Autodesk Fusion 360 part; units mm, degrees
(part 5 of 5)
sketch "Sketch25" plane through (0.7254, 0, 5.7707) normal (0.12473, 0, 0.992191) x (0, 1, 0)
  line L0 (293.4635, 73.8171) -> (293.4635, 58.6434)
  arc A0 (292.1232, 54.8991) -> (293.4635, 58.6434) centre (287.5635, 58.6434) ccw
  line L1 (292.1232, 54.8991) -> (275.8299, 35.0581)
  arc A1 (273.8014, 33.6658) -> (275.8299, 35.0581) centre (272.4102, 37.8664) ccw
  line L2 (273.8014, 33.6658) -> (261.9665, 29.7462)
  arc A2 (258.1218, 32.1079) -> (261.9665, 29.7462) centre (261.039, 32.5466) ccw
  line L3 (258.1218, 32.1079) -> (254.2531, 57.8338)
  arc A3 (256.0736, 63.8745) -> (254.2531, 57.8338) centre (261.5461, 58.9306) ccw
  line L4 (256.0736, 63.8745) -> (269.2803, 78.4929)
  arc A4 (277.0376, 80.9788) -> (269.2803, 78.4929) centre (275.3, 73.0546) ccw
  line L5 (277.0376, 80.9788) -> (289.9863, 78.1394)
  arc A5 (293.4635, 73.8171) -> (289.9863, 78.1394) centre (289.0385, 73.8171) ccw
  line L6 (230.7717, 93.4693) -> (226.5548, 85.749)
  arc A6 (222.0059, 84.0707) -> (226.5548, 85.749) centre (223.3186, 87.5166) ccw
  line L7 (222.0059, 84.0707) -> (215.7224, 86.4644)
  arc A7 (214.1574, 90.5861) -> (215.7224, 86.4644) centre (216.7726, 89.2211) ccw
  line L8 (214.1574, 90.5861) -> (217.2044, 96.4242)
  arc A8 (220.6389, 100.0016) -> (217.2044, 96.4242) centre (225.0501, 92.3293) ccw
  line L9 (220.6389, 100.0016) -> (226.4521, 103.3439)
  arc A9 (230.7073, 101.7599) -> (226.4521, 103.3439) centre (227.9225, 100.7865) ccw
  line L10 (230.7073, 101.7599) -> (231.3102, 100.0349)
  arc A10 (230.7717, 93.4693) -> (231.3102, 100.0349) centre (223.6521, 97.3581) ccw
  arc A11 (211.2158, 50.6501) -> (212.3403, 56.2234) centre (209.4758, 53.9013) ccw
  line L11 (211.2158, 50.6501) -> (201.0039, 45.1846)
  arc A12 (196.7325, 47.1438) -> (201.0039, 45.1846) centre (199.6118, 47.7855) ccw
  line L12 (196.7325, 47.1438) -> (190.7528, 73.975)
  arc A13 (195.9237, 76.4744) -> (190.7528, 73.975) centre (193.6321, 74.6167) ccw
  line L13 (195.9237, 76.4744) -> (212.3403, 56.2234)
  arc A14 (133.0891, 19.5942) -> (135.5665, 15.0427) centre (135.5665, 17.9927) ccw
  line L14 (133.0891, 19.5942) -> (153.5813, 51.294)
  arc A15 (157.3818, 52.3291) -> (153.5813, 51.294) centre (156.0587, 49.6924) ccw
  line L15 (157.3818, 52.3291) -> (171.2495, 45.3704)
  arc A16 (175.2679, 40.8003) -> (171.2495, 45.3704) centre (167.6111, 38.1196) ccw
  line L16 (175.2679, 40.8003) -> (182.9119, 18.9675)
  arc A17 (180.1276, 15.0427) -> (182.9119, 18.9675) centre (180.1276, 17.9927) ccw
  line L17 (180.1276, 15.0427) -> (135.5665, 15.0427)
  line L18 (123.35, 103.697) -> (120.1949, 82.505)
  arc A18 (115.2719, 78.7654) -> (120.1949, 82.505) centre (115.8182, 83.1566) ccw
  line L19 (115.2719, 78.7654) -> (87.1104, 82.2687)
  arc A19 (83.9707, 86.7489) -> (87.1104, 82.2687) centre (87.5657, 85.928) ccw
  line L20 (83.9707, 86.7489) -> (88.0477, 104.6024)
  arc A20 (92.2179, 107.9276) -> (88.0477, 104.6024) centre (92.2179, 103.6501) ccw
  line L21 (92.2179, 107.9276) -> (119.7027, 107.9276)
  arc A21 (123.35, 103.697) -> (119.7027, 107.9276) centre (119.7027, 104.2401) ccw
  line L22 (85.4902, 103.2388) -> (81.1941, 84.4262)
  arc A22 (79.0443, 81.4437) -> (81.1941, 84.4262) centre (76.5925, 85.477) ccw
  line L23 (79.0443, 81.4437) -> (65.0016, 72.9802)
  arc A23 (62.0516, 72.6514) -> (65.0016, 72.9802) centre (63.1527, 76.1707) ccw
  line L24 (62.0516, 72.6514) -> (12.6248, 88.1163)
  arc A24 (10.1419, 91.4948) -> (12.6248, 88.1163) centre (13.6819, 91.4948) ccw
  line L25 (10.1419, 91.4948) -> (10.1419, 100.0343)
  arc A25 (13.5344, 103.4268) -> (10.1419, 100.0343) centre (13.5344, 100.0343) ccw
  line L26 (13.5344, 103.4268) -> (37.6527, 103.4268)
  line L27 (37.6527, 103.4268) -> (42.657, 107.9276)
  line L28 (42.657, 107.9276) -> (81.7514, 107.9276)
  arc A26 (85.4902, 103.2388) -> (81.7514, 107.9276) centre (81.7514, 104.0926) ccw
  arc A27 (103.6411, 44.2546) -> (107.543, 46.9984) centre (104.5933, 47.0467) ccw
  line L29 (103.6411, 44.2546) -> (75.7593, 53.7636)
  arc A28 (71.4916, 57.5515) -> (75.7593, 53.7636) centre (78.1398, 60.7438) ccw
  line L30 (71.4916, 57.5515) -> (66.9703, 66.9675)
  arc A29 (68.665, 72.6667) -> (66.9703, 66.9675) centre (70.9592, 68.8829) ccw
  line L31 (68.665, 72.6667) -> (79.3035, 79.1172)
  arc A30 (85.3097, 80.4194) -> (79.3035, 79.1172) centre (84.1979, 71.0451) ccw
  line L32 (85.3097, 80.4194) -> (105.004, 78.0835)
  arc A31 (107.9965, 74.659) -> (105.004, 78.0835) centre (104.6045, 74.7146) ccw
  line L33 (107.9965, 74.659) -> (107.543, 46.9984)
  line L34 (77.6309, 51.2153) -> (106.5409, 41.2402)
  arc A32 (108.7653, 39.733) -> (106.5409, 41.2402) centre (104.857, 36.36) ccw
  line L35 (108.7653, 39.733) -> (125.8648, 19.9201)
  arc A33 (123.6315, 15.0427) -> (125.8648, 19.9201) centre (123.6315, 17.9927) ccw
  line L36 (123.6315, 15.0427) -> (71.6211, 15.0427)
  arc A34 (67.2556, 20.1909) -> (71.6211, 15.0427) centre (71.6211, 19.4677) ccw
  line L37 (67.2556, 20.1909) -> (71.8221, 47.7555)
  arc A35 (77.6309, 51.2153) -> (71.8221, 47.7555) centre (76.1876, 47.0323) ccw
  arc A36 (213.8317, 57.7017) -> (217.428, 56.9204) centre (216.1194, 59.5643) ccw
  line L38 (213.8317, 57.7017) -> (196.1913, 79.369)
  arc A37 (198.0965, 84.1566) -> (196.1913, 79.369) centre (198.479, 81.2315) ccw
  line L39 (198.0965, 84.1566) -> (208.6237, 85.5329)
  arc A38 (213.4569, 85.0107) -> (208.6237, 85.5329) centre (209.9622, 75.2951) ccw
  line L40 (213.4569, 85.0107) -> (222.0557, 81.9177)
  arc A39 (226.309, 78.3859) -> (222.0557, 81.9177) centre (219.3099, 74.284) ccw
  line L41 (226.309, 78.3859) -> (232.4628, 67.8857)
  arc A40 (231.2263, 63.7503) -> (232.4628, 67.8857) centre (229.9177, 66.3941) ccw
  line L42 (231.2263, 63.7503) -> (217.428, 56.9204)
  line L43 (249.3606, 15.0427) -> (236.4115, 15.0427)
  arc A41 (232.5299, 17.3431) -> (236.4115, 15.0427) centre (236.4115, 19.4677) ccw
  line L44 (232.5299, 17.3431) -> (215.1327, 49.1283)
  arc A42 (216.7158, 54.1958) -> (215.1327, 49.1283) centre (218.3674, 50.8988) ccw
  line L45 (216.7158, 54.1958) -> (232.339, 62.0219)
  arc A43 (239.2829, 63.0131) -> (232.339, 62.0219) centre (237.2937, 52.1309) ccw
  line L46 (239.2829, 63.0131) -> (248.8594, 61.2625)
  arc A44 (252.4432, 57.5422) -> (248.8594, 61.2625) centre (248.0637, 56.9097) ccw
  line L47 (252.4432, 57.5422) -> (256.3019, 30.8271)
  arc A45 (255.7697, 24.7696) -> (256.3019, 30.8271) centre (243.1633, 28.9294) ccw
  line L48 (255.7697, 24.7696) -> (253.5627, 18.0811)
  arc A46 (249.3606, 15.0427) -> (253.5627, 18.0811) centre (249.3606, 19.4677) ccw
  line L49 (293.4635, 103.5026) -> (293.4635, 84.9001)
  arc A47 (287.9958, 80.5997) -> (293.4635, 84.9001) centre (289.0385, 84.9001) ccw
  line L50 (287.9958, 80.5997) -> (274.4552, 83.8829)
  arc A48 (272.2404, 86.2656) -> (274.4552, 83.8829) centre (275.1504, 86.7498) ccw
  line L51 (272.2404, 86.2656) -> (269.4929, 102.7762)
  arc A49 (273.8579, 107.9276) -> (269.4929, 102.7762) centre (273.8579, 103.5026) ccw
  line L52 (273.8579, 107.9276) -> (289.0385, 107.9276)
  arc A50 (293.4635, 103.5026) -> (289.0385, 107.9276) centre (289.0385, 103.5026) ccw
  line L53 (290.9668, 32.2801) -> (281.6207, 33.491)
  arc A51 (280.1951, 37.0893) -> (281.6207, 33.491) centre (281.9049, 35.6851) ccw
  line L54 (280.1951, 37.0893) -> (289.5412, 48.4704)
  arc A52 (293.4635, 47.0663) -> (289.5412, 48.4704) centre (291.251, 47.0663) ccw
  arc A53 (290.9668, 32.2801) -> (293.4635, 34.4743) centre (291.251, 34.4743) ccw
  line L55 (233.851, 98.8529) -> (232.3424, 102.9719)
  arc A54 (235.8049, 107.9276) -> (232.3424, 102.9719) centre (235.8049, 104.2401) ccw
  line L56 (235.8049, 107.9276) -> (262.6115, 107.9276)
  arc A55 (266.9865, 104.166) -> (262.6115, 107.9276) centre (262.6115, 103.5026) ccw
  line L57 (266.9865, 104.166) -> (268.8676, 91.7606)
  arc A56 (264.0999, 87.6951) -> (268.8676, 91.7606) centre (265.2218, 91.2078) ccw
  line L58 (264.0999, 87.6951) -> (236.1917, 96.6084)
  arc A57 (233.851, 98.8529) -> (236.1917, 96.6084) centre (237.3135, 100.1211) ccw
  line L59 (201.7431, 17.6617) -> (199.3291, 39.0432)
  arc A58 (201.6545, 43.4497) -> (199.3291, 39.0432) centre (203.7262, 39.5396) ccw
  line L60 (201.6545, 43.4497) -> (210.1198, 47.9348)
  arc A59 (214.0829, 46.7549) -> (210.1198, 47.9348) centre (211.5009, 45.3281) ccw
  line L61 (214.0829, 46.7549) -> (229.1883, 19.4195)
  arc A60 (226.6063, 15.0427) -> (229.1883, 19.4195) centre (226.6063, 17.9927) ccw
  line L62 (226.6063, 15.0427) -> (204.6745, 15.0427)
  arc A61 (201.7431, 17.6617) -> (204.6745, 15.0427) centre (204.6745, 17.9927) ccw
  arc A62 (156.4587, 58.9806) -> (157.4975, 54.5636) centre (158.8136, 57.2038) ccw
  line L63 (156.4587, 58.9806) -> (176.5219, 85.5722)
  arc A63 (182.035, 86.864) -> (176.5219, 85.5722) centre (180.0543, 82.9071) ccw
  line L64 (182.035, 86.864) -> (183.2206, 86.2706)
  arc A64 (187.1226, 81.2581) -> (183.2206, 86.2706) centre (179.9194, 79.6756) ccw
  line L65 (187.1226, 81.2581) -> (194.4335, 47.9794)
  arc A65 (191.3482, 44.4035) -> (194.4335, 47.9794) centre (191.5522, 47.3464) ccw
  line L66 (191.3482, 44.4035) -> (178.6355, 45.2846)
  arc A66 (173.0748, 46.7985) -> (178.6355, 45.2846) centre (179.6553, 59.9993) ccw
  line L67 (173.0748, 46.7985) -> (157.4975, 54.5636)
  line L68 (121.5744, 78.7404) -> (125.6327, 105.4212)
  arc A67 (128.5492, 107.9276) -> (125.6327, 105.4212) centre (128.5492, 104.9776) ccw
  line L69 (128.5492, 107.9276) -> (172.3385, 107.9276)
  arc A68 (175.2618, 105.3735) -> (172.3385, 107.9276) centre (172.3385, 104.9776) ccw
  line L70 (175.2618, 105.3735) -> (177.1399, 91.508)
  arc A69 (176.2747, 88.2323) -> (177.1399, 91.508) centre (172.7549, 90.914) ccw
  line L71 (176.2747, 88.2323) -> (152.619, 57.1839)
  arc A70 (146.4088, 56.3524) -> (152.619, 57.1839) centre (149.0992, 59.8656) ccw
  line L72 (146.4088, 56.3524) -> (123.5394, 73.8653)
  arc A71 (121.5744, 78.7404) -> (123.5394, 73.8653) centre (126.6782, 77.9641) ccw
  line L73 (64.1302, 68.3113) -> (70.1435, 55.2951)
  arc A72 (70.492, 52.7161) -> (70.1435, 55.2951) centre (66.1265, 53.4393) ccw
  line L74 (70.492, 52.7161) -> (64.7618, 18.1275)
  arc A73 (61.1239, 15.0427) -> (64.7618, 18.1275) centre (61.1239, 18.7302) ccw
  line L75 (61.1239, 15.0427) -> (53.0443, 15.0427)
  arc A74 (50.5643, 16.3952) -> (53.0443, 15.0427) centre (53.0443, 17.9927) ccw
  line L76 (50.5643, 16.3952) -> (10.9643, 77.8757)
  arc A75 (10.1419, 80.6712) -> (10.9643, 77.8757) centre (15.3044, 80.6712) ccw
  line L77 (10.1419, 80.6712) -> (10.1419, 82.7029)
  arc A76 (13.9723, 85.5184) -> (10.1419, 82.7029) centre (13.0919, 82.7029) ccw
  line L78 (13.9723, 85.5184) -> (61.4337, 70.6789)
  arc A77 (64.1302, 68.3113) -> (61.4337, 70.6789) centre (60.1132, 66.4555) ccw
  arc A78 (10.1419, 18.7302) -> (13.8294, 15.0427) centre (13.8294, 18.7302) ccw
  line L79 (10.1419, 18.7302) -> (10.1419, 65.1989)
  arc A79 (15.5677, 66.8029) -> (10.1419, 65.1989) centre (13.0919, 65.1989) ccw
  line L80 (15.5677, 66.8029) -> (45.4146, 20.7352)
  arc A80 (42.3199, 15.0427) -> (45.4146, 20.7352) centre (42.3199, 18.7302) ccw
  line L81 (42.3199, 15.0427) -> (13.8294, 15.0427)
  arc A81 (127.0398, 21.5138) -> (131.7372, 21.8193) centre (129.273, 23.4413) ccw
  line L82 (127.0398, 21.5138) -> (111.2377, 39.8234)
  arc A82 (109.448, 44.8203) -> (111.2377, 39.8234) centre (116.8209, 44.642) ccw
  line L83 (109.448, 44.8203) -> (110.1305, 73.0437)
  arc A83 (116.5331, 76.1094) -> (110.1305, 73.0437) centre (114.1118, 72.9475) ccw
  line L84 (116.5331, 76.1094) -> (147.6751, 52.2615)
  arc A84 (148.5132, 47.3064) -> (147.6751, 52.2615) centre (145.4331, 49.3338) ccw
  line L85 (148.5132, 47.3064) -> (131.7372, 21.8193)
  arc A85 (188.1391, 86.2233) -> (194.2757, 85.4006) centre (192.6185, 96.3383) ccw
  line L86 (188.1391, 86.2233) -> (180.9121, 89.4237)
  arc A86 (179.1848, 91.7143) -> (180.9121, 89.4237) centre (182.1066, 92.1211) ccw
  line L87 (179.1848, 91.7143) -> (177.3948, 104.5708)
  arc A87 (180.3167, 107.9276) -> (177.3948, 104.5708) centre (180.3167, 104.9776) ccw
  line L88 (180.3167, 107.9276) -> (207.1787, 107.9276)
  arc A88 (209.3714, 106.951) -> (207.1787, 107.9276) centre (207.1787, 104.9776) ccw
  line L89 (209.3714, 106.951) -> (215.0822, 100.6057)
  arc A89 (215.5, 97.2583) -> (215.0822, 100.6057) centre (212.8895, 98.6322) ccw
  line L90 (215.5, 97.2583) -> (211.2519, 89.187)
  arc A90 (209.0833, 87.6442) -> (211.2519, 89.187) centre (208.6414, 90.5609) ccw
  line L91 (209.0833, 87.6442) -> (194.2757, 85.4006)
  arc A91 (181.0984, 42.9156) -> (178.1042, 38.9921) centre (180.8863, 39.9732) ccw
  line L92 (181.0984, 42.9156) -> (194.7583, 41.9308)
  arc A92 (197.4845, 39.2503) -> (194.7583, 41.9308) centre (194.5462, 38.9884) ccw
  line L93 (197.4845, 39.2503) -> (199.3562, 18.2546)
  arc A93 (196.4178, 15.0427) -> (199.3562, 18.2546) centre (196.4178, 17.9927) ccw
  line L94 (196.4178, 15.0427) -> (188.6375, 15.0427)
  arc A94 (185.8555, 17.0116) -> (188.6375, 15.0427) centre (188.6375, 17.9927) ccw
  line L95 (185.8555, 17.0116) -> (178.1042, 38.9921)
  line L96 (264.5468, 76.607) -> (254.3494, 64.7515)
  arc A95 (249.4163, 63.057) -> (254.3494, 64.7515) centre (250.4355, 68.1179) ccw
  line L97 (249.4163, 63.057) -> (238.1606, 65.3238)
  arc A96 (235.2375, 67.389) -> (238.1606, 65.3238) centre (239.0342, 69.6617) ccw
  line L98 (235.2375, 67.389) -> (228.2248, 79.1043)
  arc A97 (228.1101, 84.2056) -> (228.2248, 79.1043) centre (232.6544, 81.7558) ccw
  line L99 (228.1101, 84.2056) -> (232.6022, 92.5381)
  arc A98 (236.9767, 94.2988) -> (232.6022, 92.5381) centre (235.8481, 90.7883) ccw
  line L100 (236.9767, 94.2988) -> (263.2633, 85.8479)
  arc A99 (265.809, 82.6487) -> (263.2633, 85.8479) centre (262.1347, 82.3374) ccw
  line L101 (265.809, 82.6487) -> (265.9528, 80.9526)
  arc A100 (264.5468, 76.607) -> (265.9528, 80.9526) centre (260.0739, 80.4544) ccw
  arc A101 (255.7129, 18.0094) -> (257.7929, 15.0427) centre (257.7929, 17.2552) ccw
  line L102 (255.7129, 18.0094) -> (257.7618, 23.6594)
  arc A102 (261.9099, 27.6959) -> (257.7618, 23.6594) centre (264.0017, 21.3966) ccw
  line L103 (261.9099, 27.6959) -> (275.0229, 32.0503)
  arc A103 (276.3301, 32.1764) -> (275.0229, 32.0503) centre (275.9526, 29.2506) ccw
  line L104 (276.3301, 32.1764) -> (290.2479, 30.3805)
  arc A104 (293.4635, 26.7234) -> (290.2479, 30.3805) centre (289.776, 26.7234) ccw
  line L105 (293.4635, 26.7234) -> (293.4635, 17.9927)
  arc A105 (290.5135, 15.0427) -> (293.4635, 17.9927) centre (290.5135, 17.9927) ccw
  line L106 (290.5135, 15.0427) -> (257.7929, 15.0427)
  arc A106 (292.6499, 13.2243) -> (294.8624, 15.4368) centre (292.6499, 15.4368) ccw
  line L107 (294.8624, 31.0481) -> (294.8624, 32.9879)
  line L108 (294.8624, 32.9879) -> (294.8624, 56.7836)
  arc A107 (294.8624, 108.8182) -> (292.6499, 111.0307) centre (292.6499, 108.8182) ccw
  line L109 (292.6499, 111.0307) -> (284.2531, 111.0307)
  line L110 (284.2531, 111.0307) -> (274.007, 111.0307)
  line L111 (274.007, 111.0307) -> (270.4315, 111.0307)
  line L112 (270.4315, 111.0307) -> (265.7097, 111.0307)
  line L113 (265.7097, 111.0307) -> (261.3107, 111.0307)
  line L114 (261.3107, 111.0307) -> (250.7246, 111.0307)
  line L115 (250.7246, 111.0307) -> (234.1793, 111.0307)
  line L116 (234.1793, 111.0307) -> (215.2497, 111.0307)
  line L117 (215.2497, 111.0307) -> (213.1252, 111.0307)
  line L118 (213.1252, 111.0307) -> (199.9113, 111.0307)
  line L119 (199.9113, 111.0307) -> (198.1151, 111.0307)
  line L120 (198.1151, 111.0307) -> (180.9538, 111.0307)
  line L121 (180.9538, 111.0307) -> (178.2981, 111.0307)
  line L122 (178.2981, 111.0307) -> (163.008, 111.0307)
  line L123 (163.008, 111.0307) -> (160.0543, 111.0307)
  line L124 (160.0543, 111.0307) -> (126.4008, 111.0307)
  line L125 (126.4008, 111.0307) -> (124.6009, 111.0307)
  line L126 (124.6009, 111.0307) -> (110.3857, 111.0307)
  line L127 (110.3857, 111.0307) -> (107.4187, 111.0307)
  line L128 (107.4187, 111.0307) -> (101.9108, 111.0307)
  line L129 (101.9108, 111.0307) -> (97.1836, 111.0307)
  line L130 (97.1836, 111.0307) -> (74.0693, 111.0307)
  line L131 (74.0693, 111.0307) -> (70.9617, 111.0307)
  line L132 (70.9617, 111.0307) -> (68.0509, 111.0307)
  line L133 (68.0509, 111.0307) -> (64.5231, 111.0307)
  line L134 (64.5231, 111.0307) -> (44.1107, 111.0307)
  line L135 (44.1107, 111.0307) -> (41.8144, 111.0307)
  line L136 (41.8144, 111.0307) -> (33.0847, 111.0307)
  line L137 (33.0847, 111.0307) -> (31.0847, 111.0307)
  line L138 (31.0847, 111.0307) -> (15.0847, 111.0307)
  line L139 (15.0847, 111.0307) -> (7.3501, 111.0307)
  arc A108 (7.3501, 111.0307) -> (5.1376, 108.8182) centre (7.3501, 108.8182) ccw
  line L140 (5.1376, 100.6654) -> (5.1376, 98.4933)
  arc A109 (5.1376, 15.4368) -> (7.3501, 13.2243) centre (7.3501, 15.4368) ccw
  line L141 (7.3501, 13.2243) -> (292.6499, 13.2243)
  circle A110 centre (191.6518, 81.2581) radius 1.75
  circle A111 centre (269.3842, 84.9697) radius 1.75
  circle A112 centre (198.3819, 42.9236) radius 1.75
  circle A113 centre (152.7627, 53.9908) radius 1.75
  circle A114 centre (119.4068, 76.904) radius 1.75
  circle A115 centre (11.091, 72.0177) radius 1.75
  circle A116 centre (129.5748, 17.1372) radius 1.75
  circle A117 centre (72.5863, 52.6097) radius 1.75
  circle A118 centre (292.5805, 51.6254) radius 1.75
  circle A119 centre (234.6499, 65.0836) radius 1.75
  circle A120 centre (221.3926, 106.0047) radius 1.75
  line L142 (293.4635, 47.0663) -> (293.4635, 34.4743)
  line L143 (294.8624, 56.7836) -> (294.8624, 58.9956)
  line L144 (294.8624, 58.9956) -> (294.8624, 69.2483)
  line L145 (294.8624, 69.2483) -> (294.8624, 77.7144)
  line L146 (294.8624, 77.7144) -> (294.8624, 82.6614)
  line L147 (294.8624, 82.6614) -> (294.8624, 87.1528)
  line L148 (294.8624, 87.1528) -> (294.8624, 98.4933)
  line L149 (294.8624, 15.4368) -> (294.8624, 31.0481)
  line L150 (294.8624, 98.4933) -> (294.8624, 100.6654)
  line L151 (294.8624, 100.6654) -> (294.8624, 108.8182)
  line L152 (5.1376, 108.8182) -> (5.1376, 100.6654)
  line L153 (5.1376, 98.4933) -> (5.1376, 87.1528)
  line L154 (5.1376, 87.1528) -> (5.1376, 82.6614)
  line L155 (5.1376, 82.6614) -> (5.1376, 77.7144)
  line L156 (5.1376, 77.7144) -> (5.1376, 69.2483)
  line L157 (5.1376, 69.2483) -> (5.1376, 58.9956)
  line L158 (5.1376, 58.9956) -> (5.1376, 56.7836)
  line L159 (5.1376, 56.7836) -> (5.1376, 32.9879)
  line L160 (5.1376, 32.9879) -> (5.1376, 31.0481)
  line L161 (5.1376, 31.0481) -> (5.1376, 15.4368)
  dimension "d653" = 3.5
  constraint equal A110 A111
  constraint equal A111 A118
  constraint equal A118 A119
  constraint equal A112 A119
  constraint equal A112 A116
  constraint equal A113 A116
  constraint equal A113 A114
  constraint equal A114 A117
  constraint equal A115 A117
  constraint equal A110 A120
  measures "d653" diameter of A110
extrude "Extrude16" cut sketch "Sketch25" against normal blind 1.5 contours A110 | A111 | A112 | A113 | A114 | A115 | A116 | A117 | A118 | A119 | A120
chamfer "Chamfer2" distance 1.25 angle 45 6 edges at (-4.7873, 298.1433, 15.6118) (-59.2873, 298.2895, 30.4488) (-4.7873, 298.0437, 6.3118) (-113.7873, 298.2662, 13.0036) (-113.7873, 298.1462, 29.1549) (-59.2873, 298.31, 4.9975)
chamfer "Chamfer3" distance 1.5 angle 45 1 edges at (-4.7873, 150, 4.9975)
equation "d119 = 0.075 mm * 29.5"
equation "d120 = 3.7241020281 mm * 29.5"
equation "d121 = 10.0699999963 mm * 29.5"
equation "d122 = 0.1244091261 mm * 29.5"
equation "d124 = 0.2210304899 mm * 29.5"
equation "d125 = 0.187599032 mm * 29.5"
equation "d126 = 0.1244091261 mm * 29.5"
equation "d127 = ( 300 mm - d121 ) / 2"
equation "d429 = d428 / 2"
